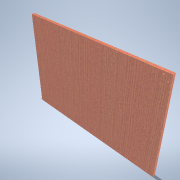
# Autodesk Inventor part: Oben
Saved by Autodesk Inventor 2021 (Build 250183000, 183)
## iProperties
Created: 2022-06-26
Part Number: Oben
Material: Holz (Birke)
Document SubType Name: Modeling
Designer: adria
Density: 0.55 g/cm^3
Appearance: Birke - natur - poliert
Mass: 3300 g
Surface Area: 7900 cm^2
Volume: 6000 cm^3
Author: adria
Autodesk Inventor part; units mm, degrees
ref_plane "YZ Plane" through (0, 0, 0) normal (1, 0, 0) x (0, 1, 0)
ref_plane "XZ Plane" through (0, 0, 0) normal (0, 1, 0) x (-1, 0, 0)
ref_plane "XY Plane" through (0, 0, 0) normal (0, 0, 1) x (1, 0, 0)
sketch "Skizze1" plane through (0, 0, 0) normal (0, 0, 1) x (1, 0, 0)
  line L0 (-375, -250) -> (375, -250)
  line L1 (375, -250) -> (375, 250)
  line L2 (375, 250) -> (-375, 250)
  line L3 (-375, 250) -> (-375, -250)
  line L4 (-375, -250) -> (375, 250) construction
  line L5 (375, -250) -> (-375, 250) construction
  point P0 (0, 0)
  dimension "d0" = 750
  dimension "d1" = 500
  constraints: 12 end point, 2 midpoint, 2 parallel, 1 horizontal, 1 perpendicular
  measures "d0" distance of L2.end L1.end
  measures "d1" distance of L1.end L0.end
extrude "Extrusion1" add sketch "Skizze1" along normal blind 16
